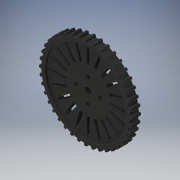
# Autodesk Inventor part: Wheel
Saved by Autodesk Inventor 2017 (Build 210142000, 142)
## iProperties
Created: 2018-02-23
Part Number: Wheel
Material: PAEK Plastic
Document SubType Name: Modeling
Designer: bradl
Density: 1.32 g/cm^3
Appearance: Rubber - Black
Author: bradl
Autodesk Inventor part; units mm, degrees
ref_plane "YZ Plane" through (0, 0, 0) normal (1, 0, 0) x (0, 1, 0)
ref_plane "XZ Plane" through (0, 0, 0) normal (0, 1, 0) x (-1, 0, 0)
ref_plane "XY Plane" through (0, 0, 0) normal (0, 0, 1) x (1, 0, 0)
sketch "Sketch2" plane through (0, 0, 0) normal (0, 0, 1) x (1, 0, 0)
  circle A0 centre (0, 0) radius 2
  line L0 (1.118, -1) -> (-1.118, -1)
  arc A1 (1.118, -1) -> (-1.118, -1) centre (0, 0) ccw
  circle A2 centre (0, 6.858) radius 1.27
  circle A3 centre (-6.858, 0) radius 1.27
  circle A4 centre (0, -6.858) radius 1.27
  circle A5 centre (6.858, 0) radius 1.27
  line L1 (-0.6088, -26.6551) -> (0.6088, -26.6551)
  line L2 (-1.5, 0) -> (-1.4967, -0.1002)
  line L3 (-0.6511, -25.3917) -> (-0.6088, -26.6551)
  line L4 (1.5, 0) -> (1.4967, -0.1002)
  line L5 (0.6511, -25.3917) -> (0.6088, -26.6551)
  line L6 (3.3291, -25.1809) -> (3.5685, -26.4222)
  line L7 (3.5685, -26.4222) -> (4.7711, -26.2317)
  line L8 (4.6152, -24.9772) -> (4.7711, -26.2317)
  line L9 (7.2273, -24.3501) -> (7.6579, -25.5386)
  line L10 (7.6579, -25.5386) -> (8.8159, -25.1624)
  line L11 (8.4656, -23.9477) -> (8.8159, -25.1624)
  line L12 (10.9475, -22.9197) -> (11.5587, -24.0263)
  line L13 (11.5587, -24.0263) -> (12.6436, -23.4735)
  line L14 (12.1077, -22.3286) -> (12.6436, -23.4735)
  line L15 (14.3981, -20.925) -> (15.1749, -21.9223)
  line L16 (15.1749, -21.9223) -> (16.16, -21.2066)
  line L17 (15.4516, -20.1596) -> (16.16, -21.2066)
  line L18 (17.4942, -18.415) -> (18.4175, -19.2785)
  line L19 (18.4175, -19.2785) -> (19.2785, -18.4175)
  line L20 (18.415, -17.4942) -> (19.2785, -18.4175)
  line L21 (20.1596, -15.4516) -> (21.2066, -16.16)
  line L22 (21.2066, -16.16) -> (21.9223, -15.1749)
  line L23 (20.925, -14.3981) -> (21.9223, -15.1749)
  line L24 (22.3286, -12.1077) -> (23.4735, -12.6436)
  line L25 (23.4735, -12.6436) -> (24.0263, -11.5587)
  line L26 (22.9197, -10.9475) -> (24.0263, -11.5587)
  line L27 (23.9477, -8.4656) -> (25.1624, -8.8159)
  line L28 (25.1624, -8.8159) -> (25.5386, -7.6579)
  line L29 (24.3501, -7.2273) -> (25.5386, -7.6579)
  line L30 (24.9772, -4.6152) -> (26.2317, -4.7711)
  line L31 (26.2317, -4.7711) -> (26.4222, -3.5685)
  line L32 (25.1809, -3.3291) -> (26.4222, -3.5685)
  line L33 (25.3917, -0.6511) -> (26.6551, -0.6088)
  line L34 (26.6551, -0.6088) -> (26.6551, 0.6088)
  line L35 (25.3917, 0.6511) -> (26.6551, 0.6088)
  line L36 (25.1809, 3.3291) -> (26.4222, 3.5685)
  line L37 (26.4222, 3.5685) -> (26.2317, 4.7711)
  line L38 (24.9772, 4.6152) -> (26.2317, 4.7711)
  line L39 (24.3501, 7.2273) -> (25.5386, 7.6579)
  line L40 (25.5386, 7.6579) -> (25.1624, 8.8159)
  line L41 (23.9477, 8.4656) -> (25.1624, 8.8159)
  line L42 (22.9197, 10.9475) -> (24.0263, 11.5587)
  line L43 (24.0263, 11.5587) -> (23.4735, 12.6436)
  line L44 (22.3286, 12.1077) -> (23.4735, 12.6436)
  line L45 (20.925, 14.3981) -> (21.9223, 15.1749)
  line L46 (21.9223, 15.1749) -> (21.2066, 16.16)
  line L47 (20.1596, 15.4516) -> (21.2066, 16.16)
  line L48 (18.415, 17.4942) -> (19.2785, 18.4175)
  line L49 (19.2785, 18.4175) -> (18.4175, 19.2785)
  line L50 (17.4942, 18.415) -> (18.4175, 19.2785)
  line L51 (15.4516, 20.1596) -> (16.16, 21.2066)
  line L52 (16.16, 21.2066) -> (15.1749, 21.9223)
  line L53 (14.3981, 20.925) -> (15.1749, 21.9223)
  line L54 (12.1077, 22.3286) -> (12.6436, 23.4735)
  line L55 (12.6436, 23.4735) -> (11.5587, 24.0263)
  line L56 (10.9475, 22.9197) -> (11.5587, 24.0263)
  line L57 (8.4656, 23.9477) -> (8.8159, 25.1624)
  line L58 (8.8159, 25.1624) -> (7.6579, 25.5386)
  line L59 (7.2273, 24.3501) -> (7.6579, 25.5386)
  line L60 (4.6152, 24.9772) -> (4.7711, 26.2317)
  line L61 (4.7711, 26.2317) -> (3.5685, 26.4222)
  line L62 (3.3291, 25.1809) -> (3.5685, 26.4222)
  line L63 (0.6511, 25.3917) -> (0.6088, 26.6551)
  line L64 (0.6088, 26.6551) -> (-0.6088, 26.6551)
  line L65 (-0.6511, 25.3917) -> (-0.6088, 26.6551)
  line L66 (-3.3291, 25.1809) -> (-3.5685, 26.4222)
  line L67 (-3.5685, 26.4222) -> (-4.7711, 26.2317)
  line L68 (-4.6152, 24.9772) -> (-4.7711, 26.2317)
  line L69 (-7.2273, 24.3501) -> (-7.6579, 25.5386)
  line L70 (-7.6579, 25.5386) -> (-8.8159, 25.1624)
  line L71 (-8.4656, 23.9477) -> (-8.8159, 25.1624)
  line L72 (-10.9475, 22.9197) -> (-11.5587, 24.0263)
  line L73 (-11.5587, 24.0263) -> (-12.6436, 23.4735)
  line L74 (-12.1077, 22.3286) -> (-12.6436, 23.4735)
  line L75 (-14.3981, 20.925) -> (-15.1749, 21.9223)
  line L76 (-15.1749, 21.9223) -> (-16.16, 21.2066)
  line L77 (-15.4516, 20.1596) -> (-16.16, 21.2066)
  line L78 (-17.4942, 18.415) -> (-18.4175, 19.2785)
  line L79 (-18.4175, 19.2785) -> (-19.2785, 18.4175)
  line L80 (-18.415, 17.4942) -> (-19.2785, 18.4175)
  line L81 (-20.1596, 15.4516) -> (-21.2066, 16.16)
  line L82 (-21.2066, 16.16) -> (-21.9223, 15.1749)
  line L83 (-20.925, 14.3981) -> (-21.9223, 15.1749)
  line L84 (-22.3286, 12.1077) -> (-23.4735, 12.6436)
  line L85 (-23.4735, 12.6436) -> (-24.0263, 11.5587)
  line L86 (-22.9197, 10.9475) -> (-24.0263, 11.5587)
  line L87 (-23.9477, 8.4656) -> (-25.1624, 8.8159)
  line L88 (-25.1624, 8.8159) -> (-25.5386, 7.6579)
  line L89 (-24.3501, 7.2273) -> (-25.5386, 7.6579)
  line L90 (-24.9772, 4.6152) -> (-26.2317, 4.7711)
  line L91 (-26.2317, 4.7711) -> (-26.4222, 3.5685)
  line L92 (-25.1809, 3.3291) -> (-26.4222, 3.5685)
  line L93 (-25.3917, 0.6511) -> (-26.6551, 0.6088)
  line L94 (-26.6551, 0.6088) -> (-26.6551, -0.6088)
  line L95 (-25.3917, -0.6511) -> (-26.6551, -0.6088)
  line L96 (-25.1809, -3.3291) -> (-26.4222, -3.5685)
  line L97 (-26.4222, -3.5685) -> (-26.2317, -4.7711)
  line L98 (-24.9772, -4.6152) -> (-26.2317, -4.7711)
  line L99 (-24.3501, -7.2273) -> (-25.5386, -7.6579)
  line L100 (-25.5386, -7.6579) -> (-25.1624, -8.8159)
  line L101 (-23.9477, -8.4656) -> (-25.1624, -8.8159)
  line L102 (-22.9197, -10.9475) -> (-24.0263, -11.5587)
  line L103 (-24.0263, -11.5587) -> (-23.4735, -12.6436)
  line L104 (-22.3286, -12.1077) -> (-23.4735, -12.6436)
  line L105 (-20.925, -14.3981) -> (-21.9223, -15.1749)
  line L106 (-21.9223, -15.1749) -> (-21.2066, -16.16)
  line L107 (-20.1596, -15.4516) -> (-21.2066, -16.16)
  line L108 (-18.415, -17.4942) -> (-19.2785, -18.4175)
  line L109 (-19.2785, -18.4175) -> (-18.4175, -19.2785)
  line L110 (-17.4942, -18.415) -> (-18.4175, -19.2785)
  line L111 (-15.4516, -20.1596) -> (-16.16, -21.2066)
  line L112 (-16.16, -21.2066) -> (-15.1749, -21.9223)
  line L113 (-14.3981, -20.925) -> (-15.1749, -21.9223)
  line L114 (-12.1077, -22.3286) -> (-12.6436, -23.4735)
  line L115 (-12.6436, -23.4735) -> (-11.5587, -24.0263)
  line L116 (-10.9475, -22.9197) -> (-11.5587, -24.0263)
  line L117 (-8.4656, -23.9477) -> (-8.8159, -25.1624)
  line L118 (-8.8159, -25.1624) -> (-7.6579, -25.5386)
  line L119 (-7.2273, -24.3501) -> (-7.6579, -25.5386)
  line L120 (-4.6152, -24.9772) -> (-4.7711, -26.2317)
  line L121 (-4.7711, -26.2317) -> (-3.5685, -26.4222)
  line L122 (-3.3291, -25.1809) -> (-3.5685, -26.4222)
  arc A6 (-3.3291, -25.1809) -> (-0.6511, -25.3917) centre (0, 0) ccw
  arc A7 (-7.2273, -24.3501) -> (-4.6152, -24.9772) centre (0, 0) ccw
  arc A8 (-10.9475, -22.9197) -> (-8.4656, -23.9477) centre (0, 0) ccw
  arc A9 (-14.3981, -20.925) -> (-12.1077, -22.3286) centre (0, 0) ccw
  arc A10 (-17.4942, -18.415) -> (-15.4516, -20.1596) centre (0, 0) ccw
  arc A11 (-20.1596, -15.4516) -> (-18.415, -17.4942) centre (0, 0) ccw
  arc A12 (-22.3286, -12.1077) -> (-20.925, -14.3981) centre (0, 0) ccw
  arc A13 (-23.9477, -8.4656) -> (-22.9197, -10.9475) centre (0, 0) ccw
  arc A14 (-24.9772, -4.6152) -> (-24.3501, -7.2273) centre (0, 0) ccw
  arc A15 (-25.3917, -0.6511) -> (-25.1809, -3.3291) centre (0, 0) ccw
  arc A16 (-25.1809, 3.3291) -> (-25.3917, 0.6511) centre (0, 0) ccw
  arc A17 (-24.3501, 7.2273) -> (-24.9772, 4.6152) centre (0, 0) ccw
  arc A18 (-22.9197, 10.9475) -> (-23.9477, 8.4656) centre (0, 0) ccw
  arc A19 (-20.925, 14.3981) -> (-22.3286, 12.1077) centre (0, 0) ccw
  arc A20 (-18.415, 17.4942) -> (-20.1596, 15.4516) centre (0, 0) ccw
  arc A21 (-15.4516, 20.1596) -> (-17.4942, 18.415) centre (0, 0) ccw
  arc A22 (-12.1077, 22.3286) -> (-14.3981, 20.925) centre (0, 0) ccw
  arc A23 (-8.4656, 23.9477) -> (-10.9475, 22.9197) centre (0, 0) ccw
  arc A24 (-4.6152, 24.9772) -> (-7.2273, 24.3501) centre (0, 0) ccw
  arc A25 (-0.6511, 25.3917) -> (-3.3291, 25.1809) centre (0, 0) ccw
  arc A26 (3.3291, 25.1809) -> (0.6511, 25.3917) centre (0, 0) ccw
  arc A27 (7.2273, 24.3501) -> (4.6152, 24.9772) centre (0, 0) ccw
  arc A28 (10.9475, 22.9197) -> (8.4656, 23.9477) centre (0, 0) ccw
  arc A29 (14.3981, 20.925) -> (12.1077, 22.3286) centre (0, 0) ccw
  arc A30 (17.4942, 18.415) -> (15.4516, 20.1596) centre (0, 0) ccw
  arc A31 (20.1596, 15.4516) -> (18.415, 17.4942) centre (0, 0) ccw
  arc A32 (0.6511, -25.3917) -> (3.3291, -25.1809) centre (0, 0) ccw
  arc A33 (4.6152, -24.9772) -> (7.2273, -24.3501) centre (0, 0) ccw
  arc A34 (8.4656, -23.9477) -> (10.9475, -22.9197) centre (0, 0) ccw
  arc A35 (12.1077, -22.3286) -> (14.3981, -20.925) centre (0, 0) ccw
  arc A36 (15.4516, -20.1596) -> (17.4942, -18.415) centre (0, 0) ccw
  arc A37 (18.415, -17.4942) -> (20.1596, -15.4516) centre (0, 0) ccw
  arc A38 (20.925, -14.3981) -> (22.3286, -12.1077) centre (0, 0) ccw
  arc A39 (22.9197, -10.9475) -> (23.9477, -8.4656) centre (0, 0) ccw
  arc A40 (24.3501, -7.2273) -> (24.9772, -4.6152) centre (0, 0) ccw
  arc A41 (25.1809, -3.3291) -> (25.3917, -0.6511) centre (0, 0) ccw
  arc A42 (25.3917, 0.6511) -> (25.1809, 3.3291) centre (0, 0) ccw
  arc A43 (24.9772, 4.6152) -> (24.3501, 7.2273) centre (0, 0) ccw
  arc A44 (23.9477, 8.4656) -> (22.9197, 10.9475) centre (0, 0) ccw
  arc A45 (22.3286, 12.1077) -> (20.925, 14.3981) centre (0, 0) ccw
  circle A46 centre (0, -6.858) radius 1.27
  circle A47 centre (-6.858, 0) radius 1.27
  circle A48 centre (0, 6.858) radius 1.27
  circle A49 centre (6.858, 0) radius 1.27
  circle A50 centre (0, 0) radius 2
  line L123 (-0.6511, -22.3616) -> (0.7541, -22.3083)
  circle A51 centre (0, 0) radius 12.7 construction
  arc A52 (-1.0196, -12.659) -> (1.0769, -12.6543) centre (0, 0) ccw
  line L124 (-1.0196, -12.659) -> (-0.6511, -22.3616)
  line L125 (1.0769, -12.6543) -> (0.7541, -22.3083)
  line L126 (-1.2487, -6.6266) -> (-1.2276, -7.1834)
  line L127 (2.9421, -12.3545) -> (6.2909, -21.4684)
  line L128 (6.2909, -21.4684) -> (7.6109, -20.9834)
  line L129 (4.9346, -11.7021) -> (7.6109, -20.9834)
  arc A53 (2.9421, -12.3545) -> (4.9346, -11.7021) centre (0, 0) ccw
  line L130 (6.6159, -10.8407) -> (12.6171, -18.4736)
  line L131 (12.6171, -18.4736) -> (13.7226, -17.6045)
  line L132 (8.3092, -9.6045) -> (13.7226, -17.6045)
  arc A54 (6.6159, -10.8407) -> (8.3092, -9.6045) centre (0, 0) ccw
  line L133 (9.642, -8.2657) -> (17.7083, -13.6706)
  line L134 (17.7083, -13.6706) -> (18.491, -12.5024)
  line L135 (10.8705, -6.5667) -> (18.491, -12.5024)
  arc A55 (9.642, -8.2657) -> (10.8705, -6.5667) centre (0, 0) ccw
  line L136 (11.7244, -4.8816) -> (21.066, -7.5293)
  line L137 (21.066, -7.5293) -> (21.4495, -6.1764)
  line L138 (12.3677, -2.8862) -> (21.4495, -6.1764)
  arc A56 (11.7244, -4.8816) -> (12.3677, -2.8862) centre (0, 0) ccw
  line L139 (12.659, -1.0196) -> (22.3616, -0.6511)
  line L140 (22.3616, -0.6511) -> (22.3083, 0.7541)
  line L141 (12.6543, 1.0769) -> (22.3083, 0.7541)
  arc A57 (12.659, -1.0196) -> (12.6543, 1.0769) centre (0, 0) ccw
  line L142 (12.3545, 2.9421) -> (21.4684, 6.2909)
  line L143 (21.4684, 6.2909) -> (20.9834, 7.6109)
  line L144 (11.7021, 4.9346) -> (20.9834, 7.6109)
  arc A58 (12.3545, 2.9421) -> (11.7021, 4.9346) centre (0, 0) ccw
  line L145 (10.8407, 6.6159) -> (18.4736, 12.6171)
  line L146 (18.4736, 12.6171) -> (17.6045, 13.7226)
  line L147 (9.6045, 8.3092) -> (17.6045, 13.7226)
  arc A59 (10.8407, 6.6159) -> (9.6045, 8.3092) centre (0, 0) ccw
  line L148 (8.2657, 9.642) -> (13.6706, 17.7083)
  line L149 (13.6706, 17.7083) -> (12.5024, 18.491)
  line L150 (6.5667, 10.8705) -> (12.5024, 18.491)
  arc A60 (8.2657, 9.642) -> (6.5667, 10.8705) centre (0, 0) ccw
  line L151 (4.8816, 11.7244) -> (7.5293, 21.066)
  line L152 (7.5293, 21.066) -> (6.1764, 21.4495)
  line L153 (2.8862, 12.3677) -> (6.1764, 21.4495)
  arc A61 (4.8816, 11.7244) -> (2.8862, 12.3677) centre (0, 0) ccw
  line L154 (1.0196, 12.659) -> (0.6511, 22.3616)
  line L155 (0.6511, 22.3616) -> (-0.7541, 22.3083)
  line L156 (-1.0769, 12.6543) -> (-0.7541, 22.3083)
  arc A62 (1.0196, 12.659) -> (-1.0769, 12.6543) centre (0, 0) ccw
  line L157 (-2.9421, 12.3545) -> (-6.2909, 21.4684)
  line L158 (-6.2909, 21.4684) -> (-7.6109, 20.9834)
  line L159 (-4.9346, 11.7021) -> (-7.6109, 20.9834)
  arc A63 (-2.9421, 12.3545) -> (-4.9346, 11.7021) centre (0, 0) ccw
  line L160 (-6.6159, 10.8407) -> (-12.6171, 18.4736)
  line L161 (-12.6171, 18.4736) -> (-13.7226, 17.6045)
  line L162 (-8.3092, 9.6045) -> (-13.7226, 17.6045)
  arc A64 (-6.6159, 10.8407) -> (-8.3092, 9.6045) centre (0, 0) ccw
  line L163 (-9.642, 8.2657) -> (-17.7083, 13.6706)
  line L164 (-17.7083, 13.6706) -> (-18.491, 12.5024)
  line L165 (-10.8705, 6.5667) -> (-18.491, 12.5024)
  arc A65 (-9.642, 8.2657) -> (-10.8705, 6.5667) centre (0, 0) ccw
  line L166 (-11.7244, 4.8816) -> (-21.066, 7.5293)
  line L167 (-21.066, 7.5293) -> (-21.4495, 6.1764)
  line L168 (-12.3677, 2.8862) -> (-21.4495, 6.1764)
  arc A66 (-11.7244, 4.8816) -> (-12.3677, 2.8862) centre (0, 0) ccw
  line L169 (-12.659, 1.0196) -> (-22.3616, 0.6511)
  line L170 (-22.3616, 0.6511) -> (-22.3083, -0.7541)
  line L171 (-12.6543, -1.0769) -> (-22.3083, -0.7541)
  arc A67 (-12.659, 1.0196) -> (-12.6543, -1.0769) centre (0, 0) ccw
  line L172 (-12.3545, -2.9421) -> (-21.4684, -6.2909)
  line L173 (-21.4684, -6.2909) -> (-20.9834, -7.6109)
  line L174 (-11.7021, -4.9346) -> (-20.9834, -7.6109)
  arc A68 (-12.3545, -2.9421) -> (-11.7021, -4.9346) centre (0, 0) ccw
  line L175 (-10.8407, -6.6159) -> (-18.4736, -12.6171)
  line L176 (-18.4736, -12.6171) -> (-17.6045, -13.7226)
  line L177 (-9.6045, -8.3092) -> (-17.6045, -13.7226)
  arc A69 (-10.8407, -6.6159) -> (-9.6045, -8.3092) centre (0, 0) ccw
  line L178 (-8.2657, -9.642) -> (-13.6706, -17.7083)
  line L179 (-13.6706, -17.7083) -> (-12.5024, -18.491)
  line L180 (-6.5667, -10.8705) -> (-12.5024, -18.491)
  arc A70 (-8.2657, -9.642) -> (-6.5667, -10.8705) centre (0, 0) ccw
  line L181 (-4.8816, -11.7244) -> (-7.5293, -21.066)
  line L182 (-7.5293, -21.066) -> (-6.1764, -21.4495)
  line L183 (-2.8862, -12.3677) -> (-6.1764, -21.4495)
  arc A71 (-4.8816, -11.7244) -> (-2.8862, -12.3677) centre (0, 0) ccw
  point P0 (0, 0)
extrude "Extrusion1" add sketch "Sketch2" along normal blind 5.334 contours L3 A6 L122 L121 L120 A7 L119 L118 L117 A8 L116 L115 L114 A9 L113 L112 L111 A10 L110 L109 L108 A11 L107 L106 L105 A12 L104 L103 L102 A13 L101 L100 L99 A14 L98 L97 L96 A15 L95 L94 L93 A16 L92 L91 L90 A17 L89 L88 L87 A18 L86 L85 L84 A19 L83 L82 L81 A20 L80 L79 L78 A21 L77 L76 L75 A22 L74 L73 L72 A23 L71 L70 L69 A24 L68 L67 L66 A25 L65 L64 L63 A26 L62 L61 L60 A27 L59 L58 L57 A28 L56 L55 L54 A29 L53 L52 L51 A30 L50 L49 L48 A31 L47 L46 L45 A45 L44 L43 L42 A44 L41 L40 L39 A43 L38 L37 L36 A42 L35 L34 L33 A41 L32 L31 L30 A40 L29 L28 L27 A39 L26 L25 L24 A38 L23 L22 L21 A37 L20 L19 L18 A36 L17 L16 L15 A35 L14 L13 L12 A34 L11 L10 L9 A33 L8 L7 L6 A32 L5 L1
sketch "Sketch3" plane through (0, 0, 5.334) normal (0, 0, 1) x (1, 0, 0)
  circle A0 centre (0, 0) radius 23.5052
  constraints: 1 centre point, 1 coincident
extrude "Extrusion2" cut sketch "Sketch3" against normal blind 1.5875
body "Solid1"
